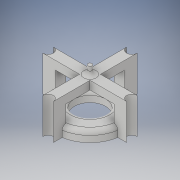
# Autodesk Inventor part: CheckValveValve1.0
Saved by Autodesk Inventor 2019 (Build 230136000, 136)
## iProperties
Created: 2019-04-04
Part Number: CheckValveValve1.0
Material: Generic
Document SubType Name: Modeling
Designer: Kepler
Density: 1 g/cm^3
Appearance: Default
Author: Kepler
Autodesk Inventor part; units mm, degrees
ref_plane "YZ Plane" through (0, 0, 0) normal (1, 0, 0) x (0, 1, 0)
ref_plane "XZ Plane" through (0, 0, 0) normal (0, 1, 0) x (-1, 0, 0)
ref_plane "XY Plane" through (0, 0, 0) normal (0, 0, 1) x (1, 0, 0)
sketch "Sketch14" plane through (0, 0, 0) normal (0, 1, 0) x (-1, 0, 0)
  arc A0 (20, 2.5) -> (20, -2.5) centre (20, 0) ccw
  arc A1 (-2.5, 20) -> (2.5, 20) centre (0, 20) ccw
  arc A2 (-20, -2.5) -> (-20, 2.5) centre (-20, 0) ccw
  arc A3 (2.5, -20) -> (-2.5, -20) centre (0, -20) ccw
  line L0 (20, -2.5) -> (15.8035, -2.5)
  line L1 (20, 2.5) -> (15.8035, 2.5)
  line L2 (2.5, 20) -> (2.5, 15.8035)
  line L3 (-2.5, 20) -> (-2.5, 15.8035)
  line L4 (-20, 2.5) -> (-15.8035, 2.5)
  line L5 (-20, -2.5) -> (-15.8035, -2.5)
  line L6 (-2.5, -20) -> (-2.5, -15.8035)
  line L7 (2.5, -20) -> (2.5, -15.8035)
  arc A4 (2.5, -15.8035) -> (15.8035, -2.5) centre (0, 0) ccw
  arc A5 (15.8035, 2.5) -> (2.5, 15.8035) centre (0, 0) ccw
  arc A6 (-2.5, 15.8035) -> (-15.8035, 2.5) centre (0, 0) ccw
  arc A7 (-15.8035, -2.5) -> (-2.5, -15.8035) centre (0, 0) ccw
  circle A8 centre (0, 0) radius 7.5
  dimension "d87" = 2.5
  dimension "d88" = 2.5
  dimension "d89" = 2.5
  dimension "d90" = 2.5
  dimension "d91" = 15
  constraints: 17 point on circle, 16 end point, 9 centre point, 4 point on line, 3 tangent, 2 coincident, 2 parallel, 1 horizontal, 1 perpendicular
  measures "d87" radius of A0
  measures "d88" radius of A1
  measures "d89" radius of A2
  measures "d90" radius of A3
  measures "d91" diameter of A8
extrude "Extrusion15" add sketch "Sketch14" along normal blind 5
sketch "Sketch15" plane through (0, 0, 0) normal (0, -1, 0) x (1, 0, 0)
  circle A0 centre (0, 0) radius 8.5
  circle A1 centre (0, 0) radius 15
  dimension "d94" = 17
  dimension "d95" = 30
  constraints: 2 centre point, 2 coincident
  measures "d94" diameter of A0
  measures "d95" diameter of A1
extrude "Extrusion16" cut sketch "Sketch15" against normal blind 1
sketch "Sketch16" plane through (0, 5, 0) normal (0, 1, 0) x (1, 0, 0)
  arc A0 (-20, -2.5) -> (-20, 2.5) centre (-20, 0) ccw projected
  arc A1 (-20, -2.5) -> (-20, 2.5) centre (-20, 0) ccw
  arc A2 (2.5, -20) -> (-2.5, -20) centre (0, -20) ccw projected
  arc A3 (2.5, -20) -> (-2.5, -20) centre (0, -20) ccw
  arc A4 (20, 2.5) -> (20, -2.5) centre (20, 0) ccw
  arc A5 (-2.5, 20) -> (2.5, 20) centre (0, 20) ccw
  line L0 (-20, 2.5) -> (-14, 2.5)
  line L1 (-14, 2.5) -> (-14, -2.5)
  line L2 (-14, -2.5) -> (-20, -2.5)
  line L3 (-2.5, -15.8035) -> (-2.5, -20) projected
  line L4 (-2.5, -20) -> (-2.5, -14)
  line L5 (-2.5, -14) -> (2.5, -14)
  line L6 (2.5, -20) -> (2.5, -15.8035) projected
  line L7 (2.5, -14) -> (2.5, -20)
  line L8 (20, -2.5) -> (14, -2.5)
  line L9 (15.8035, -2.5) -> (20, -2.5) projected
  line L10 (14, -2.5) -> (14, 2.5)
  line L11 (20, 2.5) -> (15.8035, 2.5) projected
  line L12 (14, 2.5) -> (20, 2.5)
  line L13 (2.5, 15.8035) -> (2.5, 20) projected
  line L14 (2.5, 20) -> (2.5, 14)
  line L15 (2.5, 14) -> (-2.5, 14)
  arc A6 (-2.5, 20) -> (2.5, 20) centre (0, 20) ccw projected
  line L16 (-2.5, 14) -> (-2.5, 20)
  point P0 (0, 0)
  constraints: 24 end point, 9 point on circle, 8 tangent, 7 perpendicular, 4 centre point, 4 collinear, 1 horizontal
extrude "Extrusion17" add sketch "Sketch16" along normal blind 8
sketch "Sketch17" plane through (0, 13, 0) normal (0, 1, 0) x (1, 0, 0)
  line L0 (-2.5, 20) -> (-2.5, 15.8035) projected
  arc A0 (-2.5, 20) -> (2.5, 20) centre (0, 20) ccw projected
  arc A1 (-2.5, 20) -> (2.5, 20) centre (0, 20) ccw
  arc A2 (20, 2.5) -> (20, -2.5) centre (20, 0) ccw projected
  arc A3 (20, 2.5) -> (20, -2.5) centre (20, 0) ccw
  arc A4 (2.5, -20) -> (-2.5, -20) centre (0, -20) ccw
  line L1 (-20, -2.5) -> (-2.5, -2.5)
  line L2 (-2.5, -2.5) -> (-2.5, -20)
  line L3 (2.5, -20) -> (2.5, -2.5)
  line L4 (2.5, -2.5) -> (20, -2.5)
  line L5 (20, 2.5) -> (2.5, 2.5)
  line L6 (2.5, 15.8035) -> (2.5, 20) projected
  line L7 (2.5, 2.5) -> (2.5, 20)
  line L8 (-2.5, 20) -> (-2.5, 2.5)
  line L9 (-20, 2.5) -> (-2.5, 2.5)
  arc A5 (-20, -2.5) -> (-20, 2.5) centre (-20, 0) ccw
  point P0 (0, 0)
  constraints: 16 end point, 9 point on circle, 4 centre point, 4 tangent, 3 point on line, 2 horizontal, 2 parallel, 2 perpendicular, 1 coincident, 1 collinear
extrude "Extrusion18" add sketch "Sketch17" along normal blind 4
sketch "Sketch18" plane through (0, 17, 0) normal (0, 1, 0) x (1, 0, 0)
  circle A0 centre (0, 0) radius 1
  dimension "d102" = 2
  constraints: 1 centre point, 1 coincident
  measures "d102" diameter of A0
extrude "Extrusion19" add sketch "Sketch18" along normal blind 4
fillet "Fillet1" radius 2 5 edges at (11.3137, 5, -11.3137) (7.5, 5, 0) (-11.3137, 5, -11.3137) (-11.3137, 5, 11.3137) (11.3137, 5, 11.3137)
fillet "Fillet2" radius 2 1 edges at (-1, 17, 0)
body "Solid5"
